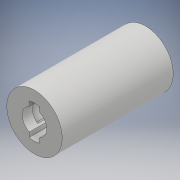
# Autodesk Inventor part: EncoderHandleSupport
Saved by Autodesk Inventor 2018 (Build 220112000, 112)
## iProperties
Created: 2019-06-17
Part Number: EncoderHandleSupport
Material: Generic
Document SubType Name: Modeling
Designer: aal_9
Density: 1 g/cm^3
Appearance: Default
Author: aal_9
Autodesk Inventor part; units mm, degrees
ref_plane "YZ Plane" through (0, 0, 0) normal (1, 0, 0) x (0, 1, 0)
ref_plane "XZ Plane" through (0, 0, 0) normal (0, 1, 0) x (-1, 0, 0)
sketch "Sketch1" plane through (0, 0, 0) normal (0, 1, 0) x (-1, 0, 0)
  circle A0 centre (0, 0) radius 10.875
  dimension "d0" = 21.75
  constraints: 1 centre point, 1 coincident
  measures "d0" diameter of A0
extrude "Extrusion1" add sketch "Sketch1" along normal blind 43.6
sketch "Sketch2" plane through (0, 0, 0) normal (0, -1, 0) x (1, 0, 0)
  circle A0 centre (0, 0) radius 2
  dimension "d3" = 4
  constraints: 1 centre point, 1 coincident
  measures "d3" diameter of A0
extrude "Extrusion2" cut sketch "Sketch2" against normal through all
sketch "Sketch3" plane through (0, 0, 0) normal (0, -1, 0) x (1, 0, 0)
  line L0 (-2, -6.1847) -> (-2, 6.1847)
  line L1 (2, 6.1847) -> (2, -6.1847)
  arc A0 (2, 6.1847) -> (-2, 6.1847) centre (0, 0) ccw
  arc A1 (-2, -6.1847) -> (2, -6.1847) centre (0, 0) ccw
  dimension "d26" = 6.5
  dimension "d27" = 4
  dimension "d28" = 2
  constraints: 4 end point, 4 point on circle, 2 centre point, 1 concentric, 1 parallel
  measures "d26" radius of A1
  measures "d27" distance between parallel lines of L0 L1
  measures "d28" distance from line of A0.centre L1
extrude "Extrusion3" cut sketch "Sketch3" against normal blind 12
sketch "Sketch4" plane through (0, 12, 0) normal (0, -1, 0) x (1, 0, 0)
  line L0 (2, -7.1361) -> (-2, -7.1361) construction
  line L1 (-2, -7.1361) -> (-2, 7.9296) construction
  line L2 (-2, 7.9296) -> (2, 7.9296) construction
  line L3 (2, 7.9296) -> (2, -7.1361) construction
  line L4 (7.1801, -1.836) -> (5.1801, -5.3001) construction
  line L5 (5.1801, -5.3001) -> (-7.8673, 2.2328) construction
  line L6 (-7.8673, 2.2328) -> (-5.8673, 5.6969) construction
  line L7 (-5.8673, 5.6969) -> (7.1801, -1.836) construction
  arc A0 (-2, 6.1847) -> (-6.3561, 1.3603) centre (0, 0) ccw
  arc A1 (2, -6.1847) -> (6.3561, -1.3603) centre (0, 0) ccw
  line L8 (-2, 6.1847) -> (-2, 3.4641)
  line L9 (6.3561, -1.3603) -> (-2, 3.4641)
  line L10 (2, -6.1847) -> (2, -3.4641)
  line L11 (2, -3.4641) -> (-6.3561, 1.3603)
  dimension "d29" = 4
  dimension "d32" = 60
  constraints: 24 end point, 8 point on line, 4 point on circle, 2 centre point, 2 collinear, 2 parallel, 1 coincident, 1 horizontal, 1 perpendicular, 10 other
  measures "d29" distance of L1.end L2.end
extrude "Extrusion4" cut sketch "Sketch4" along normal blind 4.5
ref_plane "Work Plane1" through (0, 8, 0) normal (0, -1, 0) x (1, 0, 0)
sketch "Sketch5" plane through (0, 8, 0) normal (0, -1, 0) x (1, 0, 0)
  line L0 (2, -9.381) -> (-2, -9.381) construction
  line L1 (-2, -9.381) -> (-2, 10.3615) construction
  line L2 (-2, 10.3615) -> (2, 10.3615) construction
  line L3 (2, 10.3615) -> (2, -9.381) construction
  line L4 (9.1242, -2.9584) -> (7.1242, -6.4225) construction
  line L5 (7.1242, -6.4225) -> (-9.9734, 3.4487) construction
  line L6 (-9.9734, 3.4487) -> (-7.9734, 6.9128) construction
  line L7 (-7.9734, 6.9128) -> (9.1242, -2.9584) construction
  line L8 (7.1242, 6.4225) -> (9.1242, 2.9584) construction
  line L9 (9.1242, 2.9584) -> (-7.9734, -6.9128) construction
  line L10 (-7.9734, -6.9128) -> (-9.9734, -3.4487) construction
  line L11 (-9.9734, -3.4487) -> (7.1242, 6.4225) construction
  line L12 (2, -3.4641) -> (4.3561, -4.8244)
  line L13 (2, 6.1847) -> (2, 1.1547) projected
  line L14 (0, 2.3094) -> (2, 1.1547)
  line L15 (2, 1.1547) -> (2, -3.4641)
  line L16 (-2, 3.4641) -> (-4.3561, 4.8244)
  line L17 (-2, -6.1847) -> (-2, -1.1547) projected
  line L18 (-2, 3.4641) -> (-2, -1.1547)
  line L19 (-2, -1.1547) -> (0, -2.3094)
  line L20 (-4.3561, -4.8244) -> (0, -2.3094)
  arc A0 (-4.3561, 4.8244) -> (-4.3561, -4.8244) centre (0, 0) ccw
  arc A1 (4.3561, -4.8244) -> (4.3561, 4.8244) centre (0, 0) ccw
  line L21 (0, 2.3094) -> (4.3561, 4.8244)
  dimension "d37" = 4
  dimension "d40" = 60
  dimension "d44" = 60
  constraints: 41 end point, 12 point on line, 4 point on circle, 2 centre point, 2 coincident, 2 parallel, 1 collinear, 1 horizontal, 1 perpendicular, 18 other
  measures "d37" distance of L1.end L2.end
extrude "Extrusion5" cut sketch "Sketch5" along normal blind 4
sketch "Sketch6" plane through (0, 0, 0) normal (0, -1, 0) x (1, 0, 0)
  circle A0 centre (0, 0) radius 4.8
  dimension "d49" = 9.6
  constraints: 1 centre point, 1 coincident
  measures "d49" diameter of A0
extrude "Extrusion6" cut sketch "Sketch6" against normal blind 27
sketch "Sketch7" plane through (0, 43.6, 0) normal (0, 1, 0) x (1, 0, 0)
  line L0 (0, 0) -> (8.3053, 8.3053) construction
  line L1 (0, 0) -> (11.7454, 0) construction
  point P0 (5.1265, 5.1265)
  point P1 (-5.1265, -5.1265)
  dimension "d68" = 45
  dimension "d69" = 14.5
  dimension "d70" = 7.25
  constraints: 4 end point, 1 equal length, 1 horizontal, 1 point on line
  measures "d68" angle of L1 L0
  measures "d69" distance of point (-5.127, -5.127) point (5.127, 5.127)
  measures "d70" distance of L0.start point (5.127, 5.127)
hole "Hole1" at (-5.1265, 43.6, 5.1265) at (5.1265, 43.6, -5.1265) direction (0, -1, 0) diameter 1.567 depth 5 tip angle 118 thread size "M2x0.4" class "6H" standard "ANSI Metric M Profile"
equation "\"d70\" = 0.5 * d69"
body "Solid1"
